Autodesk Inventor part; units mm, degrees
(part 2 of 3)
  spline S240 degree 2 poles (31.8228, -11.8031) (31.6251, -11.8624) (31.3137, -11.9217) (31.0715, -11.9217) knots 0 0 0 1 2 2 2
  line L303 (33.9089, -11.8179) -> (33.1377, -11.8179)
  line L304 (33.1377, -11.8179) -> (33.1377, -5.446)
  line L305 (33.1377, -5.446) -> (33.9089, -5.446)
  line L306 (33.9089, -5.446) -> (33.9089, -11.8179)
  spline S241 degree 2 poles (37.0281, -11.9217) (35.9307, -11.9217) (34.7245, -10.6908) (34.7245, -9.5539) knots 0 0 0 1 2 2 2
  spline S242 degree 2 poles (34.7245, -9.5539) (34.7245, -8.4367) (35.8961, -7.1119) (36.8403, -7.1119) knots 0 0 0 1 2 2 2
  spline S243 degree 2 poles (36.8403, -7.1119) (37.2654, -7.1119) (37.9228, -7.3591) (38.165, -7.621) knots 0 0 0 1 2 2 2
  spline S244 degree 2 poles (38.165, -7.621) (38.4122, -7.883) (38.6742, -8.6394) (38.6742, -9.1881) knots 0 0 0 1 2 2 2
  line L307 (38.6742, -9.1881) -> (38.6742, -9.6082)
  line L308 (38.6742, -9.6082) -> (35.5056, -9.6082)
  spline S245 degree 2 poles (35.5056, -9.6082) (35.5056, -10.4041) (36.3064, -11.2494) (37.0182, -11.2494) knots 0 0 0 1 2 2 2
  spline S246 degree 2 poles (37.0182, -11.2494) (37.2703, -11.2494) (37.7597, -11.1357) (37.9574, -11.0467) knots 0 0 0 1 2 2 2
  spline S247 degree 2 poles (37.9574, -11.0467) (38.165, -10.9479) (38.4518, -10.7749) (38.5457, -10.6958) knots 0 0 0 1 2 2 2
  line L309 (38.5457, -10.6958) -> (38.5902, -10.6958)
  line L310 (38.5902, -10.6958) -> (38.5902, -11.5361)
  spline S248 degree 2 poles (38.5902, -11.5361) (38.4567, -11.5905) (38.0514, -11.7487) (37.8932, -11.7932) knots 0 0 0 1 2 2 2
  spline S249 degree 2 poles (37.8932, -11.7932) (37.6707, -11.8574) (37.3049, -11.9217) (37.0281, -11.9217) knots 0 0 0 1 2 2 2
  spline S250 degree 2 poles (37.9228, -9.02) (37.9129, -8.7086) (37.7844, -8.2538) (37.6608, -8.1005) knots 0 0 0 1 2 2 2
  spline S251 degree 2 poles (37.6608, -8.1005) (37.5274, -7.9275) (37.1072, -7.7446) (36.7958, -7.7446) knots 0 0 0 1 2 2 2
  spline S252 degree 2 poles (36.7958, -7.7446) (36.4893, -7.7446) (36.0592, -7.9275) (35.8813, -8.1055) knots 0 0 0 1 2 2 2
  spline S253 degree 2 poles (35.8813, -8.1055) (35.7082, -8.2884) (35.5303, -8.7283) (35.5056, -9.02) knots 0 0 0 1 2 2 2
  line L311 (35.5056, -9.02) -> (37.9228, -9.02)
  spline S254 degree 2 poles (42.006, -11.3334) (41.9121, -11.4027) (41.5957, -11.6498) (41.4474, -11.724) knots 0 0 0 1 2 2 2
  spline S255 degree 2 poles (41.4474, -11.724) (41.2447, -11.8327) (40.8641, -11.9464) (40.518, -11.9464) knots 0 0 0 1 2 2 2
  spline S256 degree 2 poles (40.518, -11.9464) (40.2363, -11.9464) (39.7271, -11.7339) (39.5343, -11.5411) knots 0 0 0 1 2 2 2
  spline S257 degree 2 poles (39.5343, -11.5411) (39.3514, -11.3532) (39.129, -10.7996) (39.129, -10.4931) knots 0 0 0 1 2 2 2
  spline S258 degree 2 poles (39.129, -10.4931) (39.129, -10.0185) (39.5294, -9.3462) (39.9644, -9.1535) knots 0 0 0 1 2 2 2
  spline S259 degree 2 poles (39.9644, -9.1535) (40.35, -8.9755) (41.3979, -8.842) (42.006, -8.8074) knots 0 0 0 1 2 2 2
  line L312 (42.006, -8.8074) -> (42.006, -8.6591)
  spline S260 degree 2 poles (42.006, -8.6591) (42.006, -8.3922) (41.8428, -8.061) (41.6945, -7.9671) knots 0 0 0 1 2 2 2
  spline S261 degree 2 poles (41.6945, -7.9671) (41.5462, -7.8732) (41.1211, -7.8138) (40.8937, -7.8138) knots 0 0 0 1 2 2 2
  spline S262 degree 2 poles (40.8937, -7.8138) (40.6268, -7.8138) (39.9051, -7.972) (39.5442, -8.1253) knots 0 0 0 1 2 2 2
  line L313 (39.5442, -8.1253) -> (39.4997, -8.1253)
  line L314 (39.4997, -8.1253) -> (39.4997, -7.3393)
  spline S263 degree 2 poles (39.4997, -7.3393) (39.7123, -7.28) (40.5082, -7.1317) (40.8987, -7.1317) knots 0 0 0 1 2 2 2
  spline S264 degree 2 poles (40.8987, -7.1317) (41.3732, -7.1317) (42.0208, -7.28) (42.2779, -7.4727) knots 0 0 0 1 2 2 2
  spline S265 degree 2 poles (42.2779, -7.4727) (42.53, -7.6606) (42.7771, -8.2587) (42.7771, -8.6888) knots 0 0 0 1 2 2 2
  line L315 (42.7771, -8.6888) -> (42.7771, -11.8179)
  line L316 (42.7771, -11.8179) -> (42.006, -11.8179)
  line L317 (42.006, -11.8179) -> (42.006, -11.3334)
  line L318 (42.006, -10.6908) -> (42.006, -9.4204)
  spline S266 degree 2 poles (42.006, -9.4204) (41.7291, -9.4451) (40.8937, -9.5292) (40.6317, -9.6082) knots 0 0 0 1 2 2 2
  spline S267 degree 2 poles (40.6317, -9.6082) (40.3253, -9.7022) (39.9249, -10.0927) (39.9249, -10.4387) knots 0 0 0 1 2 2 2
  spline S268 degree 2 poles (39.9249, -10.4387) (39.9249, -10.8342) (40.3697, -11.2346) (40.7949, -11.2346) knots 0 0 0 1 2 2 2
  spline S269 degree 2 poles (40.7949, -11.2346) (41.1557, -11.2346) (41.7489, -10.9232) (42.006, -10.6908) knots 0 0 0 1 2 2 2
  line L319 (47.4535, -11.8179) -> (46.6823, -11.8179)
  line L320 (46.6823, -11.8179) -> (46.6823, -9.2078)
  spline S270 degree 2 poles (46.6823, -9.2078) (46.6823, -8.8915) (46.623, -8.3477) (46.534, -8.1846) knots 0 0 0 1 2 2 2
  spline S271 degree 2 poles (46.534, -8.1846) (46.4401, -8.0116) (46.1039, -7.8435) (45.8172, -7.8435) knots 0 0 0 1 2 2 2
  spline S272 degree 2 poles (45.8172, -7.8435) (45.5305, -7.8435) (44.9225, -8.15) (44.6309, -8.3971) knots 0 0 0 1 2 2 2
  line L321 (44.6309, -8.3971) -> (44.6309, -11.8179)
  line L322 (44.6309, -11.8179) -> (43.8597, -11.8179)
  line L323 (43.8597, -11.8179) -> (43.8597, -7.2404)
  line L324 (43.8597, -7.2404) -> (44.6309, -7.2404)
  line L325 (44.6309, -7.2404) -> (44.6309, -7.7496)
  spline S273 degree 2 poles (44.6309, -7.7496) (44.9769, -7.4381) (45.6442, -7.1119) (46.0199, -7.1119) knots 0 0 0 1 2 2 2
  spline S274 degree 2 poles (46.0199, -7.1119) (46.6922, -7.1119) (47.4535, -8.0017) (47.4535, -8.847) knots 0 0 0 1 2 2 2
  line L326 (47.4535, -8.847) -> (47.4535, -11.8179)
  line L327 (16.9892, -26.7663) -> (13.2274, -26.7663)
  line L328 (13.2274, -26.7663) -> (13.2274, -25.9012)
  spline S275 degree 2 poles (13.2274, -25.9012) (13.6327, -25.5206) (14.3545, -24.8137) (14.7005, -24.4331) knots 0 0 0 1 2 2 2
  spline S276 degree 2 poles (14.7005, -24.4331) (15.3975, -23.6669) (15.9067, -22.7474) (15.9067, -22.258) knots 0 0 0 1 2 2 2
  spline S277 degree 2 poles (15.9067, -22.258) (15.9067, -22.001) (15.7485, -21.6154) (15.6051, -21.4918) knots 0 0 0 1 2 2 2
  spline S278 degree 2 poles (15.6051, -21.4918) (15.4618, -21.3683) (15.0861, -21.2447) (14.8587, -21.2447) knots 0 0 0 1 2 2 2
  spline S279 degree 2 poles (14.8587, -21.2447) (14.6412, -21.2447) (14.1963, -21.3534) (13.9936, -21.4375) knots 0 0 0 1 2 2 2
  spline S280 degree 2 poles (13.9936, -21.4375) (13.8206, -21.5067) (13.4993, -21.7044) (13.4004, -21.7736) knots 0 0 0 1 2 2 2
  line L329 (13.4004, -21.7736) -> (13.3559, -21.7736)
  line L330 (13.3559, -21.7736) -> (13.3559, -20.9036)
  spline S281 degree 2 poles (13.3559, -20.9036) (13.608, -20.78) (14.5127, -20.5378) (14.918, -20.5378) knots 0 0 0 1 2 2 2
  spline S282 degree 2 poles (14.918, -20.5378) (15.7732, -20.5378) (16.7371, -21.4424) (16.7371, -22.2136) knots 0 0 0 1 2 2 2
  spline S283 degree 2 poles (16.7371, -22.2136) (16.7371, -22.5744) (16.5691, -23.1775) (16.4208, -23.4345) knots 0 0 0 1 2 2 2
  spline S284 degree 2 poles (16.4208, -23.4345) (16.2725, -23.7015) (15.8424, -24.2255) (15.6051, -24.4776) knots 0 0 0 1 2 2 2
  spline S285 degree 2 poles (15.6051, -24.4776) (15.2195, -24.8978) (14.2754, -25.7974) (13.9936, -26.0594) knots 0 0 0 1 2 2 2
  line L331 (13.9936, -26.0594) -> (16.9892, -26.0594)
  line L332 (16.9892, -26.0594) -> (16.9892, -26.7663)
  line L333 (21.7298, -24.6704) -> (21.0032, -24.6704)
  line L334 (21.0032, -24.6704) -> (21.0032, -26.7663)
  line L335 (21.0032, -26.7663) -> (20.2172, -26.7663)
  line L336 (20.2172, -26.7663) -> (20.2172, -24.6704)
  line L337 (20.2172, -24.6704) -> (17.5231, -24.6704)
  line L338 (17.5231, -24.6704) -> (17.5231, -23.8102)
  line L339 (17.5231, -23.8102) -> (20.2518, -20.6663)
  line L340 (20.2518, -20.6663) -> (21.0032, -20.6663)
  line L341 (21.0032, -20.6663) -> (21.0032, -24.0129)
  line L342 (21.0032, -24.0129) -> (21.7298, -24.0129)
  line L343 (21.7298, -24.0129) -> (21.7298, -24.6704)
  line L344 (20.2172, -24.0129) -> (20.2172, -21.6302)
  line L345 (20.2172, -21.6302) -> (18.1657, -24.0129)
  line L346 (18.1657, -24.0129) -> (20.2172, -24.0129)
  line L347 (26.9796, -20.6663) -> (24.8787, -26.7663)
  line L348 (24.8787, -26.7663) -> (24.0037, -26.7663)
  line L349 (24.0037, -26.7663) -> (21.9028, -20.6663)
  line L350 (21.9028, -20.6663) -> (22.7729, -20.6663)
  line L351 (22.7729, -20.6663) -> (24.4635, -25.7332)
  line L352 (24.4635, -25.7332) -> (26.1541, -20.6663)
  line L353 (26.1541, -20.6663) -> (26.9796, -20.6663)
  spline S286 degree 2 poles (33.9595, -24.4034) (33.9595, -25.5255) (32.872, -26.8948) (32.0514, -26.8948) knots 0 0 0 1 2 2 2
  spline S287 degree 2 poles (32.0514, -26.8948) (31.6806, -26.8948) (31.1517, -26.7119) (30.8947, -26.5538) knots 0 0 0 1 2 2 2
  line L354 (30.8947, -26.5538) -> (30.8452, -26.7663)
  line L355 (30.8452, -26.7663) -> (30.1235, -26.7663)
  line L356 (30.1235, -26.7663) -> (30.1235, -20.3944)
  line L357 (30.1235, -20.3944) -> (30.8947, -20.3944)
  line L358 (30.8947, -20.3944) -> (30.8947, -22.6683)
  spline S288 degree 2 poles (30.8947, -22.6683) (31.1863, -22.4063) (31.8635, -22.0603) (32.2936, -22.0603) knots 0 0 0 1 2 2 2
  spline S289 degree 2 poles (32.2936, -22.0603) (33.0697, -22.0603) (33.9595, -23.3011) (33.9595, -24.4034) knots 0 0 0 1 2 2 2
  spline S290 degree 2 poles (33.1636, -24.4627) (33.1636, -23.6422) (32.6644, -22.7919) (32.1107, -22.7919) knots 0 0 0 1 2 2 2
  spline S291 degree 2 poles (32.1107, -22.7919) (31.7993, -22.7919) (31.1567, -23.0885) (30.8947, -23.3159) knots 0 0 0 1 2 2 2
  line L359 (30.8947, -23.3159) -> (30.8947, -25.9408)
  spline S292 degree 2 poles (30.8947, -25.9408) (31.1863, -26.0841) (31.6362, -26.2028) (31.9031, -26.2028) knots 0 0 0 1 2 2 2
  spline S293 degree 2 poles (31.9031, -26.2028) (32.4913, -26.2028) (33.1636, -25.3674) (33.1636, -24.4627) knots 0 0 0 1 2 2 2
  line L360 (38.3195, -26.7663) -> (37.5483, -26.7663)
  line L361 (37.5483, -26.7663) -> (37.5483, -26.2621)
  spline S294 degree 2 poles (37.5483, -26.2621) (37.1924, -26.5735) (36.5547, -26.8948) (36.1592, -26.8948) knots 0 0 0 1 2 2 2
  spline S295 degree 2 poles (36.1592, -26.8948) (35.8627, -26.8948) (35.3337, -26.6971) (35.1409, -26.4845) knots 0 0 0 1 2 2 2
  spline S296 degree 2 poles (35.1409, -26.4845) (34.9432, -26.272) (34.7257, -25.6244) (34.7257, -25.1597) knots 0 0 0 1 2 2 2
  line L362 (34.7257, -25.1597) -> (34.7257, -22.1888)
  line L363 (34.7257, -22.1888) -> (35.4968, -22.1888)
  line L364 (35.4968, -22.1888) -> (35.4968, -24.7989)
  spline S297 degree 2 poles (35.4968, -24.7989) (35.4968, -25.1647) (35.5512, -25.6442) (35.6451, -25.8221) knots 0 0 0 1 2 2 2
  spline S298 degree 2 poles (35.6451, -25.8221) (35.7391, -26.0001) (36.0604, -26.1632) (36.3619, -26.1632) knots 0 0 0 1 2 2 2
  spline S299 degree 2 poles (36.3619, -26.1632) (36.6437, -26.1632) (37.2814, -25.8419) (37.5483, -25.6096) knots 0 0 0 1 2 2 2
  line L365 (37.5483, -25.6096) -> (37.5483, -22.1888)
  line L366 (37.5483, -22.1888) -> (38.3195, -22.1888)
  line L367 (38.3195, -22.1888) -> (38.3195, -26.7663)
  line L368 (40.2226, -26.7663) -> (39.4515, -26.7663)
  line L369 (39.4515, -26.7663) -> (39.4515, -20.3944)
  line L370 (39.4515, -20.3944) -> (40.2226, -20.3944)
  line L371 (40.2226, -20.3944) -> (40.2226, -26.7663)
  line L372 (45.1461, -26.7663) -> (44.1327, -26.7663)
  line L373 (44.1327, -26.7663) -> (42.4323, -24.5567)
  line L374 (42.4323, -24.5567) -> (42.1258, -24.8533)
  line L375 (42.1258, -24.8533) -> (42.1258, -26.7663)
  line L376 (42.1258, -26.7663) -> (41.3546, -26.7663)
  line L377 (41.3546, -26.7663) -> (41.3546, -20.3944)
  line L378 (41.3546, -20.3944) -> (42.1258, -20.3944)
  line L379 (42.1258, -20.3944) -> (42.1258, -24.1217)
  line L380 (42.1258, -24.1217) -> (43.935, -22.1888)
  line L381 (43.935, -22.1888) -> (44.894, -22.1888)
  line L382 (44.894, -22.1888) -> (43.0156, -24.1019)
  line L383 (43.0156, -24.1019) -> (45.1461, -26.7663)
  line L384 (-3.5915, -26.35) -> (-3.5915, -20.9717)
  line L385 (-3.5915, -20.9717) -> (-5.638, -20.9717)
  line L386 (-5.638, -20.9717) -> (-5.638, -20.25)
  line L387 (-5.638, -20.25) -> (-0.7343, -20.25)
  line L388 (-0.7343, -20.25) -> (-0.7343, -20.9717)
  line L389 (-0.7343, -20.9717) -> (-2.7808, -20.9717)
  line L390 (-2.7808, -20.9717) -> (-2.7808, -26.35)
  line L391 (-2.7808, -26.35) -> (-3.5915, -26.35)
  line L392 (3.3785, -26.35) -> (2.4343, -26.35)
  line L393 (2.4343, -26.35) -> (1.3221, -24.6297)
  line L394 (1.3221, -24.6297) -> (0.1802, -26.35)
  line L395 (0.1802, -26.35) -> (-0.6948, -26.35)
  line L396 (-0.6948, -26.35) -> (0.892, -24.081)
  line L397 (0.892, -24.081) -> (-0.6799, -21.7725)
  line L398 (-0.6799, -21.7725) -> (0.2642, -21.7725)
  line L399 (0.2642, -21.7725) -> (1.3715, -23.4779)
  line L400 (1.3715, -23.4779) -> (2.5035, -21.7725)
  line L401 (2.5035, -21.7725) -> (3.3785, -21.7725)
  line L402 (3.3785, -21.7725) -> (1.8016, -24.0316)
  line L403 (1.8016, -24.0316) -> (3.3785, -26.35)
  line L404 (0.2884, -11.9552) -> (-0.7646, -11.9552)
  line L405 (-0.7646, -11.9552) -> (-2.6924, -9.528)
  line L406 (-2.6924, -9.528) -> (-3.6218, -9.528)
  line L407 (-3.6218, -9.528) -> (-3.6218, -11.9552)
  line L408 (-3.6218, -11.9552) -> (-4.4325, -11.9552)
  line L409 (-4.4325, -11.9552) -> (-4.4325, -5.8552)
  line L410 (-4.4325, -5.8552) -> (-2.8605, -5.8552)
  spline S300 degree 2 poles (-2.8605, -5.8552) (-2.3365, -5.8552) (-1.6296, -5.9689) (-1.3083, -6.1765) knots 0 0 0 1 2 2 2
  spline S301 degree 2 poles (-1.3083, -6.1765) (-0.987, -6.3841) (-0.6163, -7.0317) (-0.6163, -7.5112) knots 0 0 0 1 2 2 2
  spline S302 degree 2 poles (-0.6163, -7.5112) (-0.6163, -8.1785) (-1.2984, -9.0832) (-1.8817, -9.3007) knots 0 0 0 1 2 2 2
  line L411 (-1.8817, -9.3007) -> (0.2884, -11.9552)
  spline S303 degree 2 poles (-1.4616, -7.5755) (-1.4616, -7.3085) (-1.6494, -6.8982) (-1.8471, -6.7648) knots 0 0 0 1 2 2 2
  spline S304 degree 2 poles (-1.8471, -6.7648) (-2.0201, -6.6511) (-2.4799, -6.5571) (-2.816, -6.5571) knots 0 0 0 1 2 2 2
  line L412 (-2.816, -6.5571) -> (-3.6218, -6.5571)
  line L413 (-3.6218, -6.5571) -> (-3.6218, -8.8508)
  line L414 (-3.6218, -8.8508) -> (-2.9099, -8.8508)
  spline S305 degree 2 poles (-2.9099, -8.8508) (-2.559, -8.8508) (-2.0004, -8.7272) (-1.8076, -8.5344) knots 0 0 0 1 2 2 2
  spline S306 degree 2 poles (-1.8076, -8.5344) (-1.6296, -8.3664) (-1.4616, -7.8918) (-1.4616, -7.5755) knots 0 0 0 1 2 2 2
  line L415 (4.2677, -11.9552) -> (3.3235, -11.9552)
  line L416 (3.3235, -11.9552) -> (2.2113, -10.2349)
  line L417 (2.2113, -10.2349) -> (1.0694, -11.9552)
  line L418 (1.0694, -11.9552) -> (0.1944, -11.9552)
  line L419 (0.1944, -11.9552) -> (1.7812, -9.6862)
  line L420 (1.7812, -9.6862) -> (0.2093, -7.3777)
  line L421 (0.2093, -7.3777) -> (1.1534, -7.3777)
  line L422 (1.1534, -7.3777) -> (2.2607, -9.0832)
  line L423 (2.2607, -9.0832) -> (3.3927, -7.3777)
  line L424 (3.3927, -7.3777) -> (4.2677, -7.3777)
  line L425 (4.2677, -7.3777) -> (2.6908, -9.6368)
  line L426 (2.6908, -9.6368) -> (4.2677, -11.9552)
  spline S307 degree 2 poles (72.332, -5.0508) (72.332, -5.4462) (72.0502, -6.1581) (71.7981, -6.4052) knots 0 0 0 1 2 2 2
  spline S308 degree 2 poles (71.7981, -6.4052) (71.4817, -6.7167) (70.6265, -7.038) (69.974, -7.038) knots 0 0 0 1 2 2 2
  line L427 (69.974, -7.038) -> (69.2869, -7.038)
  line L428 (69.2869, -7.038) -> (69.2869, -9.3119)
  line L429 (69.2869, -9.3119) -> (68.4762, -9.3119)
  line L430 (68.4762, -9.3119) -> (68.4762, -3.2119)
  line L431 (68.4762, -3.2119) -> (70.0086, -3.2119)
  spline S309 degree 2 poles (70.0086, -3.2119) (70.5524, -3.2119) (71.3136, -3.3898) (71.6053, -3.5925) knots 0 0 0 1 2 2 2
  spline S310 degree 2 poles (71.6053, -3.5925) (71.9464, -3.8249) (72.332, -4.5416) (72.332, -5.0508) knots 0 0 0 1 2 2 2
  spline S311 degree 2 poles (71.4867, -5.0755) (71.4867, -4.7591) (71.2692, -4.2945) (71.0467, -4.1462) knots 0 0 0 1 2 2 2
  spline S312 degree 2 poles (71.0467, -4.1462) (70.8539, -4.0176) (70.3398, -3.9138) (69.9592, -3.9138) knots 0 0 0 1 2 2 2
  line L432 (69.9592, -3.9138) -> (69.2869, -3.9138)
  line L433 (69.2869, -3.9138) -> (69.2869, -6.3459)
  line L434 (69.2869, -6.3459) -> (69.8405, -6.3459)
  spline S313 degree 2 poles (69.8405, -6.3459) (70.3349, -6.3459) (70.9429, -6.1877) (71.1406, -5.9801) knots 0 0 0 1 2 2 2
  spline S314 degree 2 poles (71.1406, -5.9801) (71.3235, -5.7972) (71.4867, -5.3672) (71.4867, -5.0755) knots 0 0 0 1 2 2 2
  line L435 (77.8239, -9.3119) -> (76.771, -9.3119)
  line L436 (76.771, -9.3119) -> (74.8431, -6.8847)
  line L437 (74.8431, -6.8847) -> (73.9138, -6.8847)
  line L438 (73.9138, -6.8847) -> (73.9138, -9.3119)
  line L439 (73.9138, -9.3119) -> (73.1031, -9.3119)
  line L440 (73.1031, -9.3119) -> (73.1031, -3.2119)
  line L441 (73.1031, -3.2119) -> (74.6751, -3.2119)
  spline S315 degree 2 poles (74.6751, -3.2119) (75.1991, -3.2119) (75.9059, -3.3256) (76.2273, -3.5332) knots 0 0 0 1 2 2 2
  spline S316 degree 2 poles (76.2273, -3.5332) (76.5486, -3.7408) (76.9193, -4.3884) (76.9193, -4.8679) knots 0 0 0 1 2 2 2
  spline S317 degree 2 poles (76.9193, -4.8679) (76.9193, -5.5352) (76.2371, -6.4398) (75.6538, -6.6573) knots 0 0 0 1 2 2 2
  line L442 (75.6538, -6.6573) -> (77.8239, -9.3119)
  spline S318 degree 2 poles (76.074, -4.9321) (76.074, -4.6652) (75.8862, -4.2549) (75.6884, -4.1214) knots 0 0 0 1 2 2 2
  spline S319 degree 2 poles (75.6884, -4.1214) (75.5154, -4.0078) (75.0557, -3.9138) (74.7196, -3.9138) knots 0 0 0 1 2 2 2
  line L443 (74.7196, -3.9138) -> (73.9138, -3.9138)
  line L444 (73.9138, -3.9138) -> (73.9138, -6.2075)
  line L445 (73.9138, -6.2075) -> (74.6256, -6.2075)
  spline S320 degree 2 poles (74.6256, -6.2075) (74.9766, -6.2075) (75.5352, -6.0839) (75.728, -5.8911) knots 0 0 0 1 2 2 2
  spline S321 degree 2 poles (75.728, -5.8911) (75.9059, -5.7231) (76.074, -5.2485) (76.074, -4.9321) knots 0 0 0 1 2 2 2
  spline S322 degree 2 poles (80.0089, -9.4206) (79.3465, -9.4206) (78.4171, -9.1438) (78.0068, -8.9461) knots 0 0 0 1 2 2 2
  line L446 (78.0068, -8.9461) -> (78.0068, -7.9278)
  line L447 (78.0068, -7.9278) -> (78.0662, -7.9278)
  spline S323 degree 2 poles (78.0662, -7.9278) (78.4666, -8.3035) (79.4799, -8.7187) (79.9495, -8.7187) knots 0 0 0 1 2 2 2
  spline S324 degree 2 poles (79.9495, -8.7187) (80.6218, -8.7187) (81.3089, -8.1601) (81.3089, -7.7004) knots 0 0 0 1 2 2 2
  spline S325 degree 2 poles (81.3089, -7.7004) (81.3089, -7.3346) (80.9481, -6.8798) (80.5576, -6.7661) knots 0 0 0 1 2 2 2
  spline S326 degree 2 poles (80.5576, -6.7661) (80.2758, -6.687) (79.8062, -6.5783) (79.4552, -6.4893) knots 0 0 0 1 2 2 2
  spline S327 degree 2 poles (79.4552, -6.4893) (79.1388, -6.4052) (78.6396, -6.1531) (78.4468, -5.9505) knots 0 0 0 1 2 2 2
  spline S328 degree 2 poles (78.4468, -5.9505) (78.2589, -5.7478) (78.0513, -5.204) (78.0513, -4.8481) knots 0 0 0 1 2 2 2
  spline S329 degree 2 poles (78.0513, -4.8481) (78.0513, -4.1066) (79.2081, -3.1031) (80.1028, -3.1031) knots 0 0 0 1 2 2 2
  spline S330 degree 2 poles (80.1028, -3.1031) (80.6169, -3.1031) (81.5264, -3.3058) (81.917, -3.4986) knots 0 0 0 1 2 2 2
  line L448 (81.917, -3.4986) -> (81.917, -4.4675)
  line L449 (81.917, -4.4675) -> (81.8576, -4.4675)
  spline S331 degree 2 poles (81.8576, -4.4675) (81.566, -4.2005) (80.6564, -3.8051) (80.1572, -3.8051) knots 0 0 0 1 2 2 2
  spline S332 degree 2 poles (80.1572, -3.8051) (79.5936, -3.8051) (78.8966, -4.334) (78.8966, -4.7641) knots 0 0 0 1 2 2 2
  spline S333 degree 2 poles (78.8966, -4.7641) (78.8966, -5.1496) (79.3069, -5.6094) (79.6925, -5.7132) knots 0 0 0 1 2 2 2
  spline S334 degree 2 poles (79.6925, -5.7132) (79.9495, -5.7824) (80.696, -5.9603) (80.9431, -6.0345) knots 0 0 0 1 2 2 2
  spline S335 degree 2 poles (80.9431, -6.0345) (81.5709, -6.2273) (82.1542, -7.0034) (82.1542, -7.5719) knots 0 0 0 1 2 2 2
  spline S336 degree 2 poles (82.1542, -7.5719) (82.1542, -7.9327) (81.8626, -8.6248) (81.6006, -8.867) knots 0 0 0 1 2 2 2
  spline S337 degree 2 poles (81.6006, -8.867) (81.3089, -9.1339) (80.5675, -9.4206) (80.0089, -9.4206) knots 0 0 0 1 2 2 2
  line L450 (86.2621, -9.3119) -> (83.2863, -9.3119)
  line L451 (83.2863, -9.3119) -> (83.2863, -8.689)
  line L452 (83.2863, -8.689) -> (84.3935, -8.689)
  line L453 (84.3935, -8.689) -> (84.3935, -4.6009)
  line L454 (84.3935, -4.6009) -> (83.2863, -4.6009)
  line L455 (83.2863, -4.6009) -> (83.2863, -4.0424)
  spline S338 degree 2 poles (83.2863, -4.0424) (83.9141, -4.0424) (84.5072, -3.6864) (84.5468, -3.1921) knots 0 0 0 1 2 2 2
  line L456 (84.5468, -3.1921) -> (85.1795, -3.1921)
  line L457 (85.1795, -3.1921) -> (85.1795, -8.689)
  line L458 (85.1795, -8.689) -> (86.2621, -8.689)
  line L459 (86.2621, -8.689) -> (86.2621, -9.3119)
  spline S339 degree 2 poles (91.1807, -6.2619) (91.1807, -7.9031) (90.2266, -9.4404) (89.233, -9.4404) knots 0 0 0 1 2 2 2
  spline S340 degree 2 poles (89.233, -9.4404) (88.2246, -9.4404) (87.2804, -7.8734) (87.2804, -6.2668) knots 0 0 0 1 2 2 2
  spline S341 degree 2 poles (87.2804, -6.2668) (87.2804, -4.6158) (88.2345, -3.0883) (89.233, -3.0883) knots 0 0 0 1 2 2 2
  spline S342 degree 2 poles (89.233, -3.0883) (90.2365, -3.0883) (91.1807, -4.6702) (91.1807, -6.2619) knots 0 0 0 1 2 2 2
  spline S343 degree 2 poles (90.1327, -8.1206) (90.2513, -7.819) (90.3502, -6.8897) (90.3502, -6.2619) knots 0 0 0 1 2 2 2
  spline S344 degree 2 poles (90.3502, -6.2619) (90.3502, -5.6341) (90.2513, -4.7097) (90.1277, -4.3983) knots 0 0 0 1 2 2 2
  spline S345 degree 2 poles (90.1277, -4.3983) (90.0042, -4.0868) (89.5741, -3.7655) (89.233, -3.7655) knots 0 0 0 1 2 2 2
  spline S346 degree 2 poles (89.233, -3.7655) (88.8919, -3.7655) (88.452, -4.0868) (88.3235, -4.4082) knots 0 0 0 1 2 2 2
  spline S347 degree 2 poles (88.3235, -4.4082) (88.1999, -4.7196) (88.1109, -5.6687) (88.1109, -6.2668) knots 0 0 0 1 2 2 2
  spline S348 degree 2 poles (88.1109, -6.2668) (88.1109, -6.9095) (88.19, -7.7696) (88.3185, -8.1057) knots 0 0 0 1 2 2 2
  spline S349 degree 2 poles (88.3185, -8.1057) (88.4371, -8.4221) (88.8771, -8.7632) (89.233, -8.7632) knots 0 0 0 1 2 2 2
  spline S350 degree 2 poles (89.233, -8.7632) (89.5692, -8.7632) (90.0091, -8.4419) (90.1327, -8.1206) knots 0 0 0 1 2 2 2
  line L460 (94.1961, -7.0133) -> (91.8876, -7.0133)
  line L461 (91.8876, -7.0133) -> (91.8876, -6.2718)
  line L462 (91.8876, -6.2718) -> (94.1961, -6.2718)
  line L463 (94.1961, -6.2718) -> (94.1961, -7.0133)
  spline S351 degree 2 poles (98.9564, -6.949) (98.9564, -8.0711) (97.8689, -9.4404) (97.0483, -9.4404) knots 0 0 0 1 2 2 2
  spline S352 degree 2 poles (97.0483, -9.4404) (96.6776, -9.4404) (96.1487, -9.2575) (95.8916, -9.0993) knots 0 0 0 1 2 2 2
  line L464 (95.8916, -9.0993) -> (95.8422, -9.3119)
  line L465 (95.8422, -9.3119) -> (95.1205, -9.3119)
  line L466 (95.1205, -9.3119) -> (95.1205, -2.94)
  line L467 (95.1205, -2.94) -> (95.8916, -2.94)
  line L468 (95.8916, -2.94) -> (95.8916, -5.2139)
  spline S353 degree 2 poles (95.8916, -5.2139) (96.1833, -4.9519) (96.8605, -4.6059) (97.2906, -4.6059) knots 0 0 0 1 2 2 2
  spline S354 degree 2 poles (97.2906, -4.6059) (98.0666, -4.6059) (98.9564, -5.8466) (98.9564, -6.949) knots 0 0 0 1 2 2 2
  spline S355 degree 2 poles (98.1606, -7.0083) (98.1606, -6.1877) (97.6613, -5.3375) (97.1076, -5.3375) knots 0 0 0 1 2 2 2
  spline S356 degree 2 poles (97.1076, -5.3375) (96.7962, -5.3375) (96.1536, -5.6341) (95.8916, -5.8615) knots 0 0 0 1 2 2 2
  line L469 (95.8916, -5.8615) -> (95.8916, -8.4864)
  spline S357 degree 2 poles (95.8916, -8.4864) (96.1833, -8.6297) (96.6331, -8.7484) (96.9, -8.7484) knots 0 0 0 1 2 2 2
  spline S358 degree 2 poles (96.9, -8.7484) (97.4883, -8.7484) (98.1606, -7.9129) (98.1606, -7.0083) knots 0 0 0 1 2 2 2
  spline S359 degree 2 poles (102.308, -8.8274) (102.2141, -8.8966) (101.8977, -9.1438) (101.7494, -9.218) knots 0 0 0 1 2 2 2
  spline S360 degree 2 poles (101.7494, -9.218) (101.5467, -9.3267) (101.1661, -9.4404) (100.82, -9.4404) knots 0 0 0 1 2 2 2
  spline S361 degree 2 poles (100.82, -9.4404) (100.5383, -9.4404) (100.0291, -9.2278) (99.8363, -9.0351) knots 0 0 0 1 2 2 2
  spline S362 degree 2 poles (99.8363, -9.0351) (99.6534, -8.8472) (99.431, -8.2936) (99.431, -7.9871) knots 0 0 0 1 2 2 2
  spline S363 degree 2 poles (99.431, -7.9871) (99.431, -7.5125) (99.8314, -6.8402) (100.2664, -6.6475) knots 0 0 0 1 2 2 2
  spline S364 degree 2 poles (100.2664, -6.6475) (100.652, -6.4695) (101.7, -6.336) (102.308, -6.3014) knots 0 0 0 1 2 2 2
  line L470 (102.308, -6.3014) -> (102.308, -6.1531)
  spline S365 degree 2 poles (102.308, -6.1531) (102.308, -5.8862) (102.1448, -5.555) (101.9965, -5.4611) knots 0 0 0 1 2 2 2
  spline S366 degree 2 poles (101.9965, -5.4611) (101.8482, -5.3672) (101.4231, -5.3078) (101.1957, -5.3078) knots 0 0 0 1 2 2 2
  spline S367 degree 2 poles (101.1957, -5.3078) (100.9288, -5.3078) (100.2071, -5.466) (99.8462, -5.6193) knots 0 0 0 1 2 2 2
  line L471 (99.8462, -5.6193) -> (99.8017, -5.6193)
  line L472 (99.8017, -5.6193) -> (99.8017, -4.8333)
  spline S368 degree 2 poles (99.8017, -4.8333) (100.0143, -4.774) (100.8102, -4.6257) (101.2007, -4.6257) knots 0 0 0 1 2 2 2
  spline S369 degree 2 poles (101.2007, -4.6257) (101.6752, -4.6257) (102.3228, -4.774) (102.5799, -4.9667) knots 0 0 0 1 2 2 2
  spline S370 degree 2 poles (102.5799, -4.9667) (102.832, -5.1546) (103.0791, -5.7527) (103.0791, -6.1828) knots 0 0 0 1 2 2 2
  line L473 (103.0791, -6.1828) -> (103.0791, -9.3119)
  line L474 (103.0791, -9.3119) -> (102.308, -9.3119)
  line L475 (102.308, -9.3119) -> (102.308, -8.8274)
  line L476 (102.308, -8.1848) -> (102.308, -6.9144)
  spline S371 degree 2 poles (102.308, -6.9144) (102.0311, -6.9391) (101.1957, -7.0231) (100.9337, -7.1022) knots 0 0 0 1 2 2 2
  spline S372 degree 2 poles (100.9337, -7.1022) (100.6273, -7.1962) (100.2269, -7.5867) (100.2269, -7.9327) knots 0 0 0 1 2 2 2
  spline S373 degree 2 poles (100.2269, -7.9327) (100.2269, -8.3282) (100.6717, -8.7286) (101.0969, -8.7286) knots 0 0 0 1 2 2 2
  spline S374 degree 2 poles (101.0969, -8.7286) (101.4577, -8.7286) (102.0509, -8.4172) (102.308, -8.1848) knots 0 0 0 1 2 2 2
  spline S375 degree 2 poles (105.3975, -9.4206) (104.9378, -9.4206) (104.1419, -9.1735) (103.8799, -9.0351) knots 0 0 0 1 2 2 2
  line L477 (103.8799, -9.0351) -> (103.8799, -8.17)
  line L478 (103.8799, -8.17) -> (103.9195, -8.17)
  spline S376 degree 2 poles (103.9195, -8.17) (104.0183, -8.2491) (104.2853, -8.4369) (104.5077, -8.5407) knots 0 0 0 1 2 2 2
  spline S377 degree 2 poles (104.5077, -8.5407) (104.7005, -8.6347) (105.1751, -8.7731) (105.4272, -8.7731) knots 0 0 0 1 2 2 2
  spline S378 degree 2 poles (105.4272, -8.7731) (105.6101, -8.7731) (106.0303, -8.689) (106.1291, -8.6198) knots 0 0 0 1 2 2 2
  spline S379 degree 2 poles (106.1291, -8.6198) (106.2725, -8.5259) (106.401, -8.3133) (106.401, -8.0958) knots 0 0 0 1 2 2 2
  spline S380 degree 2 poles (106.401, -8.0958) (106.401, -7.824) (106.1044, -7.5422) (105.7238, -7.4483) knots 0 0 0 1 2 2 2
  spline S381 degree 2 poles (105.7238, -7.4483) (105.5755, -7.4137) (105.1009, -7.3148) (104.8982, -7.2604) knots 0 0 0 1 2 2 2
  spline S382 degree 2 poles (104.8982, -7.2604) (104.3743, -7.1072) (103.8997, -6.4744) (103.8997, -6.0246) knots 0 0 0 1 2 2 2
  spline S383 degree 2 poles (103.8997, -6.0246) (103.8997, -5.4018) (104.834, -4.6257) (105.6051, -4.6257) knots 0 0 0 1 2 2 2
  spline S384 degree 2 poles (105.6051, -4.6257) (105.9858, -4.6257) (106.7569, -4.8135) (107.0189, -4.9569) knots 0 0 0 1 2 2 2
  line L479 (107.0189, -4.9569) -> (107.0189, -5.7824)
  line L480 (107.0189, -5.7824) -> (106.9794, -5.7824)
  spline S385 degree 2 poles (106.9794, -5.7824) (106.6828, -5.5451) (105.9611, -5.2732) (105.5903, -5.2732) knots 0 0 0 1 2 2 2
  spline S386 degree 2 poles (105.5903, -5.2732) (105.2097, -5.2732) (104.6857, -5.5945) (104.6857, -5.9159) knots 0 0 0 1 2 2 2
  spline S387 degree 2 poles (104.6857, -5.9159) (104.6857, -6.2075) (104.9971, -6.4893) (105.3431, -6.5783) knots 0 0 0 1 2 2 2
  spline S388 degree 2 poles (105.3431, -6.5783) (105.5112, -6.6227) (105.9363, -6.7117) (106.1687, -6.7661) knots 0 0 0 1 2 2 2
  spline S389 degree 2 poles (106.1687, -6.7661) (106.6729, -6.8946) (107.187, -7.4829) (107.187, -7.992) knots 0 0 0 1 2 2 2
  spline S390 degree 2 poles (107.187, -7.992) (107.187, -8.2886) (106.9547, -8.8126) (106.7273, -9.0054) knots 0 0 0 1 2 2 2
  spline S391 degree 2 poles (106.7273, -9.0054) (106.485, -9.2081) (105.8671, -9.4206) (105.3975, -9.4206) knots 0 0 0 1 2 2 2
  spline S392 degree 2 poles (109.891, -9.4157) (108.7935, -9.4157) (107.5874, -8.1848) (107.5874, -7.0479) knots 0 0 0 1 2 2 2
  spline S393 degree 2 poles (107.5874, -7.0479) (107.5874, -5.9307) (108.7589, -4.6059) (109.7031, -4.6059) knots 0 0 0 1 2 2 2
  spline S394 degree 2 poles (109.7031, -4.6059) (110.1282, -4.6059) (110.7857, -4.8531) (111.0279, -5.115) knots 0 0 0 1 2 2 2
  spline S395 degree 2 poles (111.0279, -5.115) (111.2751, -5.377) (111.5371, -6.1334) (111.5371, -6.6821) knots 0 0 0 1 2 2 2
  line L481 (111.5371, -6.6821) -> (111.5371, -7.1022)
  line L482 (111.5371, -7.1022) -> (108.3684, -7.1022)
  spline S396 degree 2 poles (108.3684, -7.1022) (108.3684, -7.8981) (109.1692, -8.7434) (109.8811, -8.7434) knots 0 0 0 1 2 2 2
  spline S397 degree 2 poles (109.8811, -8.7434) (110.1332, -8.7434) (110.6226, -8.6297) (110.8203, -8.5407) knots 0 0 0 1 2 2 2
  spline S398 degree 2 poles (110.8203, -8.5407) (111.0279, -8.4419) (111.3146, -8.2689) (111.4085, -8.1898) knots 0 0 0 1 2 2 2
  line L483 (111.4085, -8.1898) -> (111.453, -8.1898)
  line L484 (111.453, -8.1898) -> (111.453, -9.0301)
  spline S399 degree 2 poles (111.453, -9.0301) (111.3196, -9.0845) (110.9142, -9.2427) (110.756, -9.2872) knots 0 0 0 1 2 2 2
  spline S400 degree 2 poles (110.756, -9.2872) (110.5336, -9.3514) (110.1678, -9.4157) (109.891, -9.4157) knots 0 0 0 1 2 2 2
  spline S401 degree 2 poles (110.7857, -6.514) (110.7758, -6.2026) (110.6473, -5.7478) (110.5237, -5.5945) knots 0 0 0 1 2 2 2
  spline S402 degree 2 poles (110.5237, -5.5945) (110.3902, -5.4215) (109.97, -5.2386) (109.6586, -5.2386) knots 0 0 0 1 2 2 2
  spline S403 degree 2 poles (109.6586, -5.2386) (109.3521, -5.2386) (108.9221, -5.4215) (108.7441, -5.5995) knots 0 0 0 1 2 2 2
  spline S404 degree 2 poles (108.7441, -5.5995) (108.5711, -5.7824) (108.3931, -6.2223) (108.3684, -6.514) knots 0 0 0 1 2 2 2
  line L485 (108.3684, -6.514) -> (110.7857, -6.514)
  line L486 (115.8377, -9.3119) -> (115.0666, -9.3119)
  line L487 (115.0666, -9.3119) -> (115.0666, -8.8472)
  spline S405 degree 2 poles (115.0666, -8.8472) (114.8886, -8.9955) (114.6266, -9.1932) (114.4487, -9.2773) knots 0 0 0 1 2 2 2
  spline S406 degree 2 poles (114.4487, -9.2773) (114.2855, -9.3564) (113.9346, -9.4404) (113.7022, -9.4404) knots 0 0 0 1 2 2 2
  spline S407 degree 2 poles (113.7022, -9.4404) (113.3265, -9.4404) (112.6938, -9.129) (112.4713, -8.8274) knots 0 0 0 1 2 2 2
  spline S408 degree 2 poles (112.4713, -8.8274) (112.2489, -8.5259) (112.0017, -7.6361) (112.0017, -7.0578) knots 0 0 0 1 2 2 2
  spline S409 degree 2 poles (112.0017, -7.0578) (112.0017, -6.4547) (112.3132, -5.5748) (112.585, -5.2436) knots 0 0 0 1 2 2 2
  spline S410 degree 2 poles (112.585, -5.2436) (112.8371, -4.947) (113.544, -4.6059) (113.9346, -4.6059) knots 0 0 0 1 2 2 2
  spline S411 degree 2 poles (113.9346, -4.6059) (114.2756, -4.6059) (114.7848, -4.7591) (115.0666, -4.9173) knots 0 0 0 1 2 2 2
  line L488 (115.0666, -4.9173) -> (115.0666, -2.94)
  line L489 (115.0666, -2.94) -> (115.8377, -2.94)
  line L490 (115.8377, -2.94) -> (115.8377, -9.3119)
  line L491 (115.0666, -8.1996) -> (115.0666, -5.555)
  spline S412 degree 2 poles (115.0666, -5.555) (114.7799, -5.4166) (114.3251, -5.3128) (114.0631, -5.3128) knots 0 0 0 1 2 2 2
  spline S413 degree 2 poles (114.0631, -5.3128) (113.4699, -5.3128) (112.7976, -6.2026) (112.7976, -7.0429) knots 0 0 0 1 2 2 2
  spline S414 degree 2 poles (112.7976, -7.0429) (112.7976, -7.8536) (113.3117, -8.7088) (113.8802, -8.7088) knots 0 0 0 1 2 2 2
  spline S415 degree 2 poles (113.8802, -8.7088) (114.1817, -8.7088) (114.7947, -8.432) (115.0666, -8.1996) knots 0 0 0 1 2 2 2
  line L492 (122.002, -5.5599) -> (121.9624, -5.5599)
  spline S416 degree 2 poles (121.9624, -5.5599) (121.8735, -5.5352) (121.6807, -5.5253) (121.5472, -5.5253) knots 0 0 0 1 2 2 2
  spline S417 degree 2 poles (121.5472, -5.5253) (121.2358, -5.5253) (120.6228, -5.7972) (120.346, -6.0642) knots 0 0 0 1 2 2 2
  line L493 (120.346, -6.0642) -> (120.346, -9.3119)
  line L494 (120.346, -9.3119) -> (119.5748, -9.3119)
  line L495 (119.5748, -9.3119) -> (119.5748, -4.7344)
  line L496 (119.5748, -4.7344) -> (120.346, -4.7344)
  line L497 (120.346, -4.7344) -> (120.346, -5.4166)
  spline S418 degree 2 poles (120.346, -5.4166) (120.7662, -5.0409) (121.394, -4.7344) (121.6906, -4.7344) knots 0 0 0 1 2 2 2
  spline S419 degree 2 poles (121.6906, -4.7344) (121.8092, -4.7344) (121.9278, -4.7443) (122.002, -4.7591) knots 0 0 0 1 2 2 2
  line L498 (122.002, -4.7591) -> (122.002, -5.5599)
  spline S420 degree 2 poles (124.5873, -9.4157) (123.4899, -9.4157) (122.2837, -8.1848) (122.2837, -7.0479) knots 0 0 0 1 2 2 2
  spline S421 degree 2 poles (122.2837, -7.0479) (122.2837, -5.9307) (123.4553, -4.6059) (124.3995, -4.6059) knots 0 0 0 1 2 2 2
  spline S422 degree 2 poles (124.3995, -4.6059) (124.8246, -4.6059) (125.482, -4.8531) (125.7243, -5.115) knots 0 0 0 1 2 2 2
  spline S423 degree 2 poles (125.7243, -5.115) (125.9714, -5.377) (126.2334, -6.1334) (126.2334, -6.6821) knots 0 0 0 1 2 2 2
  line L499 (126.2334, -6.6821) -> (126.2334, -7.1022)
  line L500 (126.2334, -7.1022) -> (123.0648, -7.1022)
  spline S424 degree 2 poles (123.0648, -7.1022) (123.0648, -7.8981) (123.8656, -8.7434) (124.5774, -8.7434) knots 0 0 0 1 2 2 2
  spline S425 degree 2 poles (124.5774, -8.7434) (124.8295, -8.7434) (125.3189, -8.6297) (125.5166, -8.5407) knots 0 0 0 1 2 2 2
  spline S426 degree 2 poles (125.5166, -8.5407) (125.7243, -8.4419) (126.011, -8.2689) (126.1049, -8.1898) knots 0 0 0 1 2 2 2
  line L501 (126.1049, -8.1898) -> (126.1494, -8.1898)
  line L502 (126.1494, -8.1898) -> (126.1494, -9.0301)
  spline S427 degree 2 poles (126.1494, -9.0301) (126.0159, -9.0845) (125.6106, -9.2427) (125.4524, -9.2872) knots 0 0 0 1 2 2 2
  spline S428 degree 2 poles (125.4524, -9.2872) (125.2299, -9.3514) (124.8641, -9.4157) (124.5873, -9.4157) knots 0 0 0 1 2 2 2
  spline S429 degree 2 poles (125.482, -6.514) (125.4722, -6.2026) (125.3436, -5.7478) (125.22, -5.5945) knots 0 0 0 1 2 2 2
  spline S430 degree 2 poles (125.22, -5.5945) (125.0866, -5.4215) (124.6664, -5.2386) (124.355, -5.2386) knots 0 0 0 1 2 2 2
  spline S431 degree 2 poles (124.355, -5.2386) (124.0485, -5.2386) (123.6184, -5.4215) (123.4405, -5.5995) knots 0 0 0 1 2 2 2
  spline S432 degree 2 poles (123.4405, -5.5995) (123.2675, -5.7824) (123.0895, -6.2223) (123.0648, -6.514) knots 0 0 0 1 2 2 2
  line L503 (123.0648, -6.514) -> (125.482, -6.514)
  line L504 (129.4218, -3.6815) -> (129.3823, -3.6815)
  spline S433 degree 2 poles (129.3823, -3.6815) (129.2785, -3.6419) (128.8929, -3.5727) (128.7397, -3.5727) knots 0 0 0 1 2 2 2
  spline S434 degree 2 poles (128.7397, -3.5727) (128.2552, -3.5727) (127.84, -4.0078) (127.84, -4.5812) knots 0 0 0 1 2 2 2
  line L505 (127.84, -4.5812) -> (127.84, -4.7344)
  line L506 (127.84, -4.7344) -> (129.1153, -4.7344)
  line L507 (129.1153, -4.7344) -> (129.1153, -5.3721)
  line L508 (129.1153, -5.3721) -> (127.8647, -5.3721)
  line L509 (127.8647, -5.3721) -> (127.8647, -9.3119)
  line L510 (127.8647, -9.3119) -> (127.0935, -9.3119)
  line L511 (127.0935, -9.3119) -> (127.0935, -5.3721)
  line L512 (127.0935, -5.3721) -> (126.5745, -5.3721)
  line L513 (126.5745, -5.3721) -> (126.5745, -4.7344)
  line L514 (126.5745, -4.7344) -> (127.0935, -4.7344)
  line L515 (127.0935, -4.7344) -> (127.0935, -4.5812)
  spline S435 degree 2 poles (127.0935, -4.5812) (127.0935, -3.7606) (127.8894, -2.9005) (128.6309, -2.9005) knots 0 0 0 1 2 2 2
  spline S436 degree 2 poles (128.6309, -2.9005) (128.8435, -2.9005) (129.2538, -2.9449) (129.4218, -2.9746) knots 0 0 0 1 2 2 2
  line L516 (129.4218, -2.9746) -> (129.4218, -3.6815)
  spline S437 degree 2 poles (131.671, -9.4157) (130.5736, -9.4157) (129.3675, -8.1848) (129.3675, -7.0479) knots 0 0 0 1 2 2 2
  spline S438 degree 2 poles (129.3675, -7.0479) (129.3675, -5.9307) (130.539, -4.6059) (131.4832, -4.6059) knots 0 0 0 1 2 2 2
  spline S439 degree 2 poles (131.4832, -4.6059) (131.9083, -4.6059) (132.5658, -4.8531) (132.808, -5.115) knots 0 0 0 1 2 2 2
  spline S440 degree 2 poles (132.808, -5.115) (133.0551, -5.377) (133.3171, -6.1334) (133.3171, -6.6821) knots 0 0 0 1 2 2 2
  line L517 (133.3171, -6.6821) -> (133.3171, -7.1022)
  line L518 (133.3171, -7.1022) -> (130.1485, -7.1022)
  spline S441 degree 2 poles (130.1485, -7.1022) (130.1485, -7.8981) (130.9493, -8.7434) (131.6611, -8.7434) knots 0 0 0 1 2 2 2
  spline S442 degree 2 poles (131.6611, -8.7434) (131.9132, -8.7434) (132.4026, -8.6297) (132.6004, -8.5407) knots 0 0 0 1 2 2 2
  spline S443 degree 2 poles (132.6004, -8.5407) (132.808, -8.4419) (133.0947, -8.2689) (133.1886, -8.1898) knots 0 0 0 1 2 2 2
  line L519 (133.1886, -8.1898) -> (133.2331, -8.1898)
  line L520 (133.2331, -8.1898) -> (133.2331, -9.0301)
  spline S444 degree 2 poles (133.2331, -9.0301) (133.0996, -9.0845) (132.6943, -9.2427) (132.5361, -9.2872) knots 0 0 0 1 2 2 2
  spline S445 degree 2 poles (132.5361, -9.2872) (132.3136, -9.3514) (131.9478, -9.4157) (131.671, -9.4157) knots 0 0 0 1 2 2 2
  spline S446 degree 2 poles (132.5658, -6.514) (132.5559, -6.2026) (132.4273, -5.7478) (132.3038, -5.5945) knots 0 0 0 1 2 2 2
  spline S447 degree 2 poles (132.3038, -5.5945) (132.1703, -5.4215) (131.7501, -5.2386) (131.4387, -5.2386) knots 0 0 0 1 2 2 2
  spline S448 degree 2 poles (131.4387, -5.2386) (131.1322, -5.2386) (130.7021, -5.4215) (130.5242, -5.5995) knots 0 0 0 1 2 2 2
  spline S449 degree 2 poles (130.5242, -5.5995) (130.3512, -5.7824) (130.1732, -6.2223) (130.1485, -6.514) knots 0 0 0 1 2 2 2
  line L521 (130.1485, -6.514) -> (132.5658, -6.514)
  line L522 (136.5253, -5.5599) -> (136.4858, -5.5599)
  spline S450 degree 2 poles (136.4858, -5.5599) (136.3968, -5.5352) (136.204, -5.5253) (136.0705, -5.5253) knots 0 0 0 1 2 2 2
  spline S451 degree 2 poles (136.0705, -5.5253) (135.7591, -5.5253) (135.1461, -5.7972) (134.8693, -6.0642) knots 0 0 0 1 2 2 2
  line L523 (134.8693, -6.0642) -> (134.8693, -9.3119)
  line L524 (134.8693, -9.3119) -> (134.0982, -9.3119)
  line L525 (134.0982, -9.3119) -> (134.0982, -4.7344)
  line L526 (134.0982, -4.7344) -> (134.8693, -4.7344)
  line L527 (134.8693, -4.7344) -> (134.8693, -5.4166)
  spline S452 degree 2 poles (134.8693, -5.4166) (135.2895, -5.0409) (135.9173, -4.7344) (136.2139, -4.7344) knots 0 0 0 1 2 2 2
  spline S453 degree 2 poles (136.2139, -4.7344) (136.3325, -4.7344) (136.4512, -4.7443) (136.5253, -4.7591) knots 0 0 0 1 2 2 2
  line L528 (136.5253, -4.7591) -> (136.5253, -5.5599)
  spline S454 degree 2 poles (139.1106, -9.4157) (138.0132, -9.4157) (136.8071, -8.1848) (136.8071, -7.0479) knots 0 0 0 1 2 2 2
  spline S455 degree 2 poles (136.8071, -7.0479) (136.8071, -5.9307) (137.9786, -4.6059) (138.9228, -4.6059) knots 0 0 0 1 2 2 2
  spline S456 degree 2 poles (138.9228, -4.6059) (139.3479, -4.6059) (140.0054, -4.8531) (140.2476, -5.115) knots 0 0 0 1 2 2 2
  spline S457 degree 2 poles (140.2476, -5.115) (140.4948, -5.377) (140.7568, -6.1334) (140.7568, -6.6821) knots 0 0 0 1 2 2 2
  line L529 (140.7568, -6.6821) -> (140.7568, -7.1022)
  line L530 (140.7568, -7.1022) -> (137.5881, -7.1022)
  spline S458 degree 2 poles (137.5881, -7.1022) (137.5881, -7.8981) (138.3889, -8.7434) (139.1008, -8.7434) knots 0 0 0 1 2 2 2
  spline S459 degree 2 poles (139.1008, -8.7434) (139.3529, -8.7434) (139.8423, -8.6297) (140.04, -8.5407) knots 0 0 0 1 2 2 2
  spline S460 degree 2 poles (140.04, -8.5407) (140.2476, -8.4419) (140.5343, -8.2689) (140.6282, -8.1898) knots 0 0 0 1 2 2 2
  line L531 (140.6282, -8.1898) -> (140.6727, -8.1898)
  line L532 (140.6727, -8.1898) -> (140.6727, -9.0301)
  spline S461 degree 2 poles (140.6727, -9.0301) (140.5393, -9.0845) (140.1339, -9.2427) (139.9757, -9.2872) knots 0 0 0 1 2 2 2
  spline S462 degree 2 poles (139.9757, -9.2872) (139.7533, -9.3514) (139.3875, -9.4157) (139.1106, -9.4157) knots 0 0 0 1 2 2 2
  spline S463 degree 2 poles (140.0054, -6.514) (139.9955, -6.2026) (139.867, -5.7478) (139.7434, -5.5945) knots 0 0 0 1 2 2 2
  spline S464 degree 2 poles (139.7434, -5.5945) (139.6099, -5.4215) (139.1897, -5.2386) (138.8783, -5.2386) knots 0 0 0 1 2 2 2
  spline S465 degree 2 poles (138.8783, -5.2386) (138.5718, -5.2386) (138.1418, -5.4215) (137.9638, -5.5995) knots 0 0 0 1 2 2 2
  spline S466 degree 2 poles (137.9638, -5.5995) (137.7908, -5.7824) (137.6128, -6.2223) (137.5881, -6.514) knots 0 0 0 1 2 2 2
  line L533 (137.5881, -6.514) -> (140.0054, -6.514)
  line L534 (145.1316, -9.3119) -> (144.3604, -9.3119)
  line L535 (144.3604, -9.3119) -> (144.3604, -6.7018)
  spline S467 degree 2 poles (144.3604, -6.7018) (144.3604, -6.3855) (144.3011, -5.8417) (144.2121, -5.6786) knots 0 0 0 1 2 2 2
  spline S468 degree 2 poles (144.2121, -5.6786) (144.1182, -5.5056) (143.782, -5.3375) (143.4953, -5.3375) knots 0 0 0 1 2 2 2
  spline S469 degree 2 poles (143.4953, -5.3375) (143.2086, -5.3375) (142.6006, -5.644) (142.3089, -5.8911) knots 0 0 0 1 2 2 2
  line L536 (142.3089, -5.8911) -> (142.3089, -9.3119)
  line L537 (142.3089, -9.3119) -> (141.5378, -9.3119)
  line L538 (141.5378, -9.3119) -> (141.5378, -4.7344)
  line L539 (141.5378, -4.7344) -> (142.3089, -4.7344)
  line L540 (142.3089, -4.7344) -> (142.3089, -5.2436)
  spline S470 degree 2 poles (142.3089, -5.2436) (142.655, -4.9321) (143.3223, -4.6059) (143.698, -4.6059) knots 0 0 0 1 2 2 2
  spline S471 degree 2 poles (143.698, -4.6059) (144.3703, -4.6059) (145.1316, -5.4957) (145.1316, -6.341) knots 0 0 0 1 2 2 2
  line L541 (145.1316, -6.341) -> (145.1316, -9.3119)
  spline S472 degree 2 poles (148.0333, -9.4157) (147.5587, -9.4157) (146.7727, -9.124) (146.491, -8.8274) knots 0 0 0 1 2 2 2
  spline S473 degree 2 poles (146.491, -8.8274) (146.2092, -8.5358) (145.8978, -7.6361) (145.8978, -7.033) knots 0 0 0 1 2 2 2
  spline S474 degree 2 poles (145.8978, -7.033) (145.8978, -6.43) (146.2191, -5.5501) (146.491, -5.2535) knots 0 0 0 1 2 2 2
  spline S475 degree 2 poles (146.491, -5.2535) (146.7628, -4.9519) (147.5686, -4.6306) (148.0333, -4.6306) knots 0 0 0 1 2 2 2
  spline S476 degree 2 poles (148.0333, -4.6306) (148.4089, -4.6306) (149.1109, -4.8432) (149.3828, -4.9816) knots 0 0 0 1 2 2 2
  line L542 (149.3828, -4.9816) -> (149.3828, -5.8466)
  line L543 (149.3828, -5.8466) -> (149.3383, -5.8466)
  spline S477 degree 2 poles (149.3383, -5.8466) (149.2542, -5.7774) (148.9972, -5.5995) (148.8143, -5.5056) knots 0 0 0 1 2 2 2
  spline S478 degree 2 poles (148.8143, -5.5056) (148.6512, -5.4265) (148.2162, -5.3029) (148.0184, -5.3029) knots 0 0 0 1 2 2 2
  spline S479 degree 2 poles (148.0184, -5.3029) (147.4203, -5.3029) (146.6936, -6.2075) (146.6936, -7.033) knots 0 0 0 1 2 2 2
  spline S480 degree 2 poles (146.6936, -7.033) (146.6936, -7.8388) (147.3956, -8.7434) (148.0184, -8.7434) knots 0 0 0 1 2 2 2
  spline S481 degree 2 poles (148.0184, -8.7434) (148.3941, -8.7434) (149.0763, -8.432) (149.3383, -8.1898) knots 0 0 0 1 2 2 2
  line L544 (149.3383, -8.1898) -> (149.3828, -8.1898)
  line L545 (149.3828, -8.1898) -> (149.3828, -9.0548)
  spline S482 degree 2 poles (149.3828, -9.0548) (149.2691, -9.1092) (148.923, -9.2625) (148.7846, -9.2971) knots 0 0 0 1 2 2 2
  spline S483 degree 2 poles (148.7846, -9.2971) (148.5869, -9.3564) (148.2755, -9.4157) (148.0333, -9.4157) knots 0 0 0 1 2 2 2
  spline S484 degree 2 poles (152.0719, -9.4157) (150.9745, -9.4157) (149.7683, -8.1848) (149.7683, -7.0479) knots 0 0 0 1 2 2 2
  spline S485 degree 2 poles (149.7683, -7.0479) (149.7683, -5.9307) (150.9399, -4.6059) (151.8841, -4.6059) knots 0 0 0 1 2 2 2
  spline S486 degree 2 poles (151.8841, -4.6059) (152.3092, -4.6059) (152.9666, -4.8531) (153.2089, -5.115) knots 0 0 0 1 2 2 2
  spline S487 degree 2 poles (153.2089, -5.115) (153.456, -5.377) (153.718, -6.1334) (153.718, -6.6821) knots 0 0 0 1 2 2 2
  line L546 (153.718, -6.6821) -> (153.718, -7.1022)
  line L547 (153.718, -7.1022) -> (150.5494, -7.1022)
  spline S488 degree 2 poles (150.5494, -7.1022) (150.5494, -7.8981) (151.3502, -8.7434) (152.062, -8.7434) knots 0 0 0 1 2 2 2
  spline S489 degree 2 poles (152.062, -8.7434) (152.3141, -8.7434) (152.8035, -8.6297) (153.0012, -8.5407) knots 0 0 0 1 2 2 2
  spline S490 degree 2 poles (153.0012, -8.5407) (153.2089, -8.4419) (153.4956, -8.2689) (153.5895, -8.1898) knots 0 0 0 1 2 2 2
  line L548 (153.5895, -8.1898) -> (153.634, -8.1898)
  line L549 (153.634, -8.1898) -> (153.634, -9.0301)
  spline S491 degree 2 poles (153.634, -9.0301) (153.5005, -9.0845) (153.0952, -9.2427) (152.937, -9.2872) knots 0 0 0 1 2 2 2
  spline S492 degree 2 poles (152.937, -9.2872) (152.7145, -9.3514) (152.3487, -9.4157) (152.0719, -9.4157) knots 0 0 0 1 2 2 2
  spline S493 degree 2 poles (152.9666, -6.514) (152.9568, -6.2026) (152.8282, -5.7478) (152.7047, -5.5945) knots 0 0 0 1 2 2 2
  spline S494 degree 2 poles (152.7047, -5.5945) (152.5712, -5.4215) (152.151, -5.2386) (151.8396, -5.2386) knots 0 0 0 1 2 2 2
  spline S495 degree 2 poles (151.8396, -5.2386) (151.5331, -5.2386) (151.103, -5.4215) (150.9251, -5.5995) knots 0 0 0 1 2 2 2
  spline S496 degree 2 poles (150.9251, -5.5995) (150.7521, -5.7824) (150.5741, -6.2223) (150.5494, -6.514) knots 0 0 0 1 2 2 2
  line L550 (150.5494, -6.514) -> (152.9666, -6.514)
  spline S497 degree 2 poles (158.9381, -9.4157) (158.4636, -9.4157) (157.6776, -9.124) (157.3958, -8.8274) knots 0 0 0 1 2 2 2
  spline S498 degree 2 poles (157.3958, -8.8274) (157.1141, -8.5358) (156.8026, -7.6361) (156.8026, -7.033) knots 0 0 0 1 2 2 2
  spline S499 degree 2 poles (156.8026, -7.033) (156.8026, -6.43) (157.1239, -5.5501) (157.3958, -5.2535) knots 0 0 0 1 2 2 2
  spline S500 degree 2 poles (157.3958, -5.2535) (157.6677, -4.9519) (158.4735, -4.6306) (158.9381, -4.6306) knots 0 0 0 1 2 2 2
  spline S501 degree 2 poles (158.9381, -4.6306) (159.3138, -4.6306) (160.0158, -4.8432) (160.2876, -4.9816) knots 0 0 0 1 2 2 2
  line L551 (160.2876, -4.9816) -> (160.2876, -5.8466)
  line L552 (160.2876, -5.8466) -> (160.2431, -5.8466)
  spline S502 degree 2 poles (160.2431, -5.8466) (160.1591, -5.7774) (159.9021, -5.5995) (159.7192, -5.5056) knots 0 0 0 1 2 2 2
  spline S503 degree 2 poles (159.7192, -5.5056) (159.556, -5.4265) (159.121, -5.3029) (158.9233, -5.3029) knots 0 0 0 1 2 2 2
  spline S504 degree 2 poles (158.9233, -5.3029) (158.3252, -5.3029) (157.5985, -6.2075) (157.5985, -7.033) knots 0 0 0 1 2 2 2
  spline S505 degree 2 poles (157.5985, -7.033) (157.5985, -7.8388) (158.3004, -8.7434) (158.9233, -8.7434) knots 0 0 0 1 2 2 2
  spline S506 degree 2 poles (158.9233, -8.7434) (159.299, -8.7434) (159.9812, -8.432) (160.2431, -8.1898) knots 0 0 0 1 2 2 2
  line L553 (160.2431, -8.1898) -> (160.2876, -8.1898)
  line L554 (160.2876, -8.1898) -> (160.2876, -9.0548)
  spline S507 degree 2 poles (160.2876, -9.0548) (160.1739, -9.1092) (159.8279, -9.2625) (159.6895, -9.2971) knots 0 0 0 1 2 2 2
  spline S508 degree 2 poles (159.6895, -9.2971) (159.4918, -9.3564) (159.1803, -9.4157) (158.9381, -9.4157) knots 0 0 0 1 2 2 2
  line L555 (161.7756, -9.3119) -> (161.0044, -9.3119)
  line L556 (161.0044, -9.3119) -> (161.0044, -2.94)
  line L557 (161.0044, -2.94) -> (161.7756, -2.94)
  line L558 (161.7756, -2.94) -> (161.7756, -9.3119)
  spline S509 degree 2 poles (166.6694, -7.0231) (166.6694, -8.1799) (165.5572, -9.4404) (164.6278, -9.4404) knots 0 0 0 1 2 2 2
  spline S510 degree 2 poles (164.6278, -9.4404) (163.6738, -9.4404) (162.5813, -8.1403) (162.5813, -7.0231) knots 0 0 0 1 2 2 2
  spline S511 degree 2 poles (162.5813, -7.0231) (162.5813, -5.8763) (163.7084, -4.6059) (164.6278, -4.6059) knots 0 0 0 1 2 2 2
  spline S512 degree 2 poles (164.6278, -4.6059) (165.5572, -4.6059) (166.6694, -5.8714) (166.6694, -7.0231) knots 0 0 0 1 2 2 2
  spline S513 degree 2 poles (165.8735, -7.0231) (165.8735, -6.1334) (165.226, -5.2683) (164.6278, -5.2683) knots 0 0 0 1 2 2 2
  spline S514 degree 2 poles (164.6278, -5.2683) (164.0297, -5.2683) (163.3772, -6.1334) (163.3772, -7.0231) knots 0 0 0 1 2 2 2
  spline S515 degree 2 poles (163.3772, -7.0231) (163.3772, -7.8882) (164.0297, -8.778) (164.6278, -8.778) knots 0 0 0 1 2 2 2
  spline S516 degree 2 poles (164.6278, -8.778) (165.221, -8.778) (165.8735, -7.9031) (165.8735, -7.0231) knots 0 0 0 1 2 2 2
  spline S517 degree 2 poles (169.2794, -9.4157) (168.8049, -9.4157) (168.0189, -9.124) (167.7371, -8.8274) knots 0 0 0 1 2 2 2
  spline S518 degree 2 poles (167.7371, -8.8274) (167.4554, -8.5358) (167.144, -7.6361) (167.144, -7.033) knots 0 0 0 1 2 2 2
  spline S519 degree 2 poles (167.144, -7.033) (167.144, -6.43) (167.4653, -5.5501) (167.7371, -5.2535) knots 0 0 0 1 2 2 2
  spline S520 degree 2 poles (167.7371, -5.2535) (168.009, -4.9519) (168.8148, -4.6306) (169.2794, -4.6306) knots 0 0 0 1 2 2 2
  spline S521 degree 2 poles (169.2794, -4.6306) (169.6551, -4.6306) (170.3571, -4.8432) (170.629, -4.9816) knots 0 0 0 1 2 2 2
  line L559 (170.629, -4.9816) -> (170.629, -5.8466)
  line L560 (170.629, -5.8466) -> (170.5845, -5.8466)
  spline S522 degree 2 poles (170.5845, -5.8466) (170.5004, -5.7774) (170.2434, -5.5995) (170.0605, -5.5056) knots 0 0 0 1 2 2 2
  spline S523 degree 2 poles (170.0605, -5.5056) (169.8974, -5.4265) (169.4624, -5.3029) (169.2646, -5.3029) knots 0 0 0 1 2 2 2